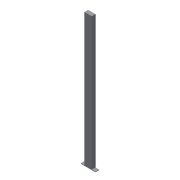
# Autodesk Inventor part: Lift Towers
Saved by Autodesk Inventor 2015 (Build 190159000, 159)
## iProperties
Created: 2015-03-07
Part Number: Lift Towers
Material: Generic
Document SubType Name: Modeling
Designer: Jaden
Density: 1 g/cm^3
Appearance: Default
Author: Jaden
Autodesk Inventor part; units mm, degrees
ref_plane "YZ Plane" through (0, 0, 0) normal (1, 0, 0) x (0, 1, 0)
ref_plane "XZ Plane" through (0, 0, 0) normal (0, 1, 0) x (-1, 0, 0)
ref_plane "XY Plane" through (0, 0, 0) normal (0, 0, 1) x (1, 0, 0)
sketch "Sketch1" plane through (0, 0, 0) normal (0, 0, 1) x (1, 0, 0)
  point P0 (0, 0)
sketch "Sketch2" plane through (0, 0, 0) normal (0, 0, 1) x (1, 0, 0)
  line L0 (0, 0) -> (-25.4, 0)
  line L1 (-25.4, 0) -> (-25.4, 3.175)
  line L2 (-25.4, 3.175) -> (0, 3.175)
  line L3 (0, 3.175) -> (0, 917.575)
  line L4 (0, 917.575) -> (50.8, 917.575)
  line L5 (50.8, 917.575) -> (50.8, 3.175)
  line L6 (50.8, 3.175) -> (76.2, 3.175)
  line L7 (76.2, 3.175) -> (76.2, 0)
  line L8 (76.2, 0) -> (0, 0)
  dimension "d0" = 25.4
  dimension "d1" = 3.175
  dimension "d2" = 914.4
  dimension "d3" = 90
  dimension "d4" = 50.8
  dimension "d5" = 90
  dimension "d6" = 25.4
  constraints: 18 end point, 5 perpendicular, 2 horizontal, 1 vertical
  measures "d0" distance of L0.start L0.end
  measures "d1" distance of L0.end L1.end
  measures "d2" distance of L2.end L3.end
  measures "d3" angle of L3 L2
  measures "d4" distance of L3.end L4.end
  measures "d5" angle of L4 L5
  measures "d6" distance of L5.end L6.end
extrude "Extrusion1" add sketch "Sketch2" along normal blind 25.4
body "Solid1"
